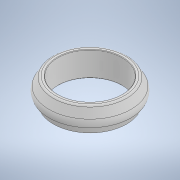
# Autodesk Inventor part: idl-tire
Saved by Autodesk Inventor 2020 (Build 240168000, 168)
## iProperties
Created: 2020-10-09
Part Number: idl-tire
Material: Generic
Document SubType Name: Modeling
Designer: alnwlsn
Density: 1 g/cm^3
Appearance: Default
Author: alnwlsn
Autodesk Inventor part; units mm, degrees
ref_plane "YZ Plane" through (0, 0, 0) normal (1, 0, 0) x (0, 1, 0)
ref_plane "XZ Plane" through (0, 0, 0) normal (0, 1, 0) x (-1, 0, 0)
ref_plane "XY Plane" through (0, 0, 0) normal (0, 0, 1) x (1, 0, 0)
sketch "Sketch1" plane through (0, 0, 0) normal (0, 0, 1) x (1, 0, 0)
  line L0 (0, 0) -> (6.45, 0)
  line L1 (6.45, 0) -> (6.45, 5)
  line L2 (6.45, 5) -> (6.9597, 5)
  line L3 (7.3939, 4.7479) -> (8.2527, 3.2437)
  line L4 (8.2527, 1.7563) -> (7.3939, 0.2521)
  line L5 (6.9597, 0) -> (6.45, 0)
  arc A0 (8.2527, 1.7563) -> (8.2527, 3.2437) centre (6.95, 2.5) ccw
  arc A1 (7.3939, 4.7479) -> (6.9597, 5) centre (6.9597, 4.5) ccw
  arc A2 (6.9597, 0) -> (7.3939, 0.2521) centre (6.9597, 0.5) ccw
  line L6 (0, 0) -> (0, 12.2617)
  point P0 (7.25, 5)
  point P1 (7.25, 0)
  dimension "d0" = 5
  dimension "d1" = 6.45
  dimension "d2" = 0.8
  dimension "d3" = 1.5
  dimension "d4" = 0.5
  dimension "d5" = 2
  constraints: 14 end point, 6 point on circle, 6 tangent, 5 point on line, 3 centre point, 2 equal length, 2 perpendicular, 1 collinear, 1 equal radius, 1 horizontal, 1 vertical
  measures "d0" distance of L0.end L1.end
  measures "d1" distance of L0.start L0.end
  measures "d2" distance of L1.end point (7.25, 5)
  measures "d3" radius of A0
  measures "d4" radius of A1
revolve "Revolution1" add sketch "Sketch1" angle 360 about axis through (0, 0, 0) along (0, 1, 0)
chamfer "Chamfer1" distance 0.1 angle 45 2 edges at (-6.45, 0, 0) (-6.45, 5, 0)
body "Solid1"
